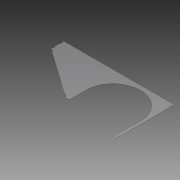
# Autodesk Inventor part: Top
Saved by Autodesk Inventor 2013 (Build 170138000, 138)
## iProperties
Created: 2013-01-27
Part Number: Top
Material: Polycarbonate, Clear
Document SubType Name: Modeling
Designer: Andrew Toennies
Density: 1.2 g/cm^3
Mass: 224.295 g
Surface Area: 1239.09 cm^2
Volume: 186.913 cm^3
Author: Andrew Toennies
Autodesk Inventor part; units mm, degrees
ref_plane "YZ Plane" through (0, 0, 0) normal (1, 0, 0) x (0, 1, 0)
ref_plane "XZ Plane" through (0, 0, 0) normal (0, 1, 0) x (-1, 0, 0)
ref_plane "XY Plane" through (0, 0, 0) normal (0, 0, 1) x (1, 0, 0)
sketch "Sketch1" plane through (0, 0, 0) normal (0, 1, 0) x (-1, 0, 0)
  line L0 (0, 0) -> (558.8, 0)
  line L1 (0, 292.1) -> (0, 0)
  arc A0 (9.525, 158.75) -> (288.925, 158.75) centre (149.225, 158.75) ccw
  line L2 (288.925, 158.75) -> (288.925, 241.3)
  line L3 (9.525, 158.75) -> (9.525, 292.1)
  line L4 (0, 292.1) -> (9.525, 292.1)
  line L5 (288.925, 241.3) -> (305.8191, 241.3)
  line L6 (558.8, 0) -> (558.8, 63.5)
  line L7 (558.8, 63.5) -> (305.8191, 241.3)
  point P0 (297.372, 241.3)
  dimension "d0" = 558.8
  dimension "d3" = 279.4
  dimension "d4" = 149.225
  dimension "d10" = 292.1
  dimension "d14" = 63.5
  constraints: 16 end point, 3 perpendicular, 2 horizontal, 2 parallel, 2 point on circle, 2 tangent, 1 centre point, 1 midpoint, 1 other
  measures "d0" distance of L0.start L0.end
  measures "d3" diameter of A0
  measures "d4" distance from line of A0.centre L1
  measures "d10" distance between parallel lines of L0 L4
  measures "d14" distance of L0.end L6.end
extrude "Extrusion2" add sketch "Sketch1" along normal blind 3.175
sketch "Sketch2" plane through (-558.8, 0, 0) normal (-1, 0, 0) x (0, 0, 1)
  line L0 (0, 0) -> (63.5, 0) projected
  line L1 (63.5, 0) -> (63.5, 3.175) projected
  line L2 (0, 3.175) -> (63.5, 3.175) projected
  line L3 (0, 0) -> (0, 3.175) projected
  line L4 (6.35, 0) -> (6.35, 3.175)
  line L5 (19.05, 3.175) -> (19.05, 0)
  line L6 (57.15, 3.175) -> (57.15, 0)
  line L7 (44.45, 3.175) -> (44.45, 0)
  dimension "d15" = 6.35
  dimension "d16" = 12.7
  dimension "d17" = 12.7
  dimension "d18" = 6.35
  constraints: 8 end point, 8 point on line, 3 perpendicular, 1 parallel
  measures "d15" distance between parallel lines of L3 L4
  measures "d16" distance between parallel lines of L5 L4
  measures "d17" distance between parallel lines of L6 L7
  measures "d18" distance between parallel lines of L1 L6
extrude "Extrusion3" cut sketch "Sketch2" against normal blind 3.175 contours L4 L2 L5 L0 | L7 L2 L6 L0
sketch "Sketch3" plane through (-558.8, 0, 63.5) normal (-0.5750096, 0, 0.8181467) x (0.8181467, 0, 0.5750096)
  line L0 (0, 0) -> (309.2122, 0) projected
  line L1 (309.2122, 0) -> (309.2122, 3.175) projected
  line L2 (0, 3.175) -> (309.2122, 3.175) projected
  line L3 (0, 0) -> (0, 3.175) projected
  line L4 (6.35, 0) -> (6.35, 3.175)
  line L5 (19.05, 3.175) -> (19.05, 0)
  line L6 (302.8622, 3.175) -> (302.8622, 0)
  line L7 (290.1622, 3.175) -> (290.1622, 0)
  point P0 (420.6672, 0)
  dimension "d21" = 12.7
  dimension "d22" = 6.35
  dimension "d23" = 6.35
  dimension "d24" = 12.7
  constraints: 8 end point, 8 point on line, 4 perpendicular
  measures "d21" distance between parallel lines of L6 L7
  measures "d22" distance between parallel lines of L1 L6
  measures "d23" distance between parallel lines of L4 L3
  measures "d24" distance between parallel lines of L5 L4
extrude "Extrusion4" cut sketch "Sketch3" against normal blind 3.175 contours L4 L2 L5 L0 | L7 L2 L6 L0
sketch "Sketch4" plane through (0, 0, 292.1) normal (1, 0, 0) x (0, 0, -1)
  line L0 (0, 0) -> (292.1, 0) projected
  line L1 (292.1, 0) -> (292.1, 3.175) projected
  line L2 (0, 3.175) -> (292.1, 3.175) projected
  line L3 (285.75, 3.175) -> (285.75, 0)
  line L4 (273.05, 3.175) -> (273.05, 0)
  line L5 (6.35, 3.175) -> (6.35, 0)
  line L6 (19.05, 3.175) -> (19.05, 0)
  dimension "d27" = 12.7
  dimension "d28" = 12.7
  dimension "d29" = 6.35
  dimension "d30" = 254
  constraints: 8 end point, 8 point on line, 3 perpendicular, 1 parallel
  measures "d27" distance between parallel lines of L6 L5
  measures "d28" distance between parallel lines of L4 L3
  measures "d29" distance between parallel lines of L1 L3
  measures "d30" distance between parallel lines of L6 L4
extrude "Extrusion5" cut sketch "Sketch4" against normal blind 3.175 contours L5 L2 L6 L0 | L4 L2 L3 L0
body "Solid2"
